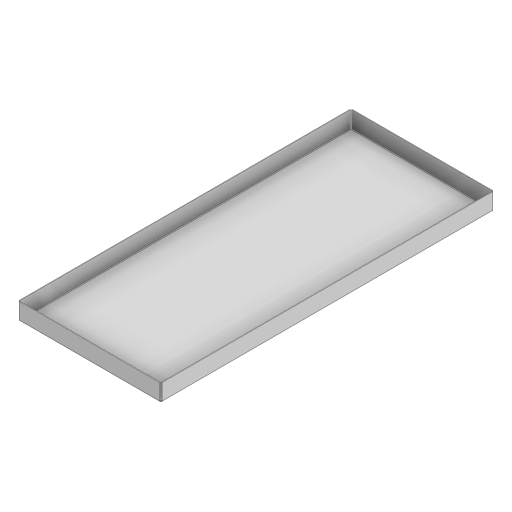
# Autodesk Inventor part: Front_plate
Saved by Autodesk Inventor 2024.2 (Build 282272000, 272)
## iProperties
Created: 2025-01-06
Part Number: Front_plate
Material: Generic
Document SubType Name: Sheet Metal
Designer: Kartik
Mass: 67.0584 g
Surface Area: 1686.48 cm^2
Volume: 67.0584 cm^3
Density: 1 g/cm^3
Sheet Metal Rule: Default_mm
Appearance: Default
Author: Kartik
Autodesk Inventor part; units mm, degrees
note: some values were not read from the file. Chosen so that the rebuilt part matches the saved one: corner form of "Plate2".
ref_plane "YZ Plane" through (0, 0, 0) normal (1, 0, 0) x (0, 1, 0)
ref_plane "XZ Plane" through (0, 0, 0) normal (0, 1, 0) x (-1, 0, 0)
ref_plane "XY Plane" through (0, 0, 0) normal (0, 0, 1) x (1, 0, 0)
sketch "Sketch1" plane through (0, 0, 0) normal (0, 1, 0) x (-1, 0, 0)
  line L0 (72.3629, 154.3951) -> (-92.6371, 154.3951)
  line L1 (-92.6371, 154.3951) -> (-92.6371, -230.4049)
  line L2 (-92.6371, -230.4049) -> (72.3629, -230.4049)
  line L3 (72.3629, -230.4049) -> (72.3629, 154.3951)
  point P0 (0, 0)
  dimension "d0" = 165
  dimension "d1" = 384.8
  measures "d0" distance of L0.start L0.end
  measures "d1" distance of L2.end L0.start
extrude "Plate1" add sketch "Sketch1" along normal blind 0.8
sketch "Sketch2" plane through (92.6371, 0, 153.5951) normal (0, 0, 1) x (1, 0, 0)
  line L0 (-165, 0) -> (0, 0)
  line L1 (0, 0) -> (0, 20)
  line L2 (0, 20) -> (-165, 20)
  line L3 (-165, 20) -> (-165, 0)
  constraints: 6 end point, 1 horizontal, 1 perpendicular, 1 vertical
edge flange "Flange1" height 20 angle 90 thickness 0.8 bend radius 0.8 thickness toward (0, 0, 1) relief tear relief width 0.8 relief depth 0.4 corner gap 0.8 corner form 2 edges at (10.1371, 0.8, 154.3951) (-72.3629, 0.8, -38.0049) (92.6371, 0.8, -38.0049) (10.1371, 0.8, -230.4049) wall of the first edge with corners at (-72.3629, 0, 153.5951) (92.6371, 0, 153.5951) (92.6371, 20, 153.5951) (-72.3629, 20, 153.5951)
bend "Bend1"
corner "Corner1"
equation "\"d2\" = Thickness"
equation "\"d3\" = BendReliefWidth"
equation "\"d4\" = BendReliefDepth"
equation "\"d5\" = MinimumRemnant"
equation "\"d6\" = TransitionRadius"
equation "\"d9\" = BendRadius"
equation "\"d10\" = CornerReliefSize"
equation "\"d11\" = GapSize"
equation "\"d12\" = JacobiRadiusSize"
equation "\"BendRadius\" = Thickness"
equation "\"BendReliefWidth\" = Thickness"
equation "\"BendReliefDepth\" = 0.5 * Thickness"
equation "\"CornerReliefSize\" = 4 * Thickness"
equation "\"MinimumRemnant\" = 2 * Thickness"
equation "\"TransitionRadius\" = BendRadius"
equation "\"JacobiRadiusSize\" = BendRadius"
equation "\"GapSize\" = Thickness"
equation "\"Thickness\" = 0.8"
body "Solid1"
